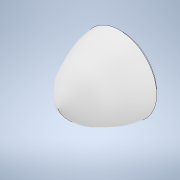
# Autodesk Inventor part: nose
Saved by Autodesk Inventor 2020 (Build 240168000, 168)
## iProperties
Created: 2021-01-23
Part Number: nose
Material: ABS Plastic
Document SubType Name: Modeling
Designer: 0x6f736f646f
Density: 1.06 g/cm^3
Appearance: Smooth - White
Author: 0x6f736f646f
Autodesk Inventor part; units mm, degrees
ref_plane "YZ Plane" through (0, 0, 0) normal (1, 0, 0) x (0, 1, 0)
ref_plane "XZ Plane" through (0, 0, 0) normal (0, 1, 0) x (-1, 0, 0)
ref_plane "XY Plane" through (0, 0, 0) normal (0, 0, 1) x (1, 0, 0)
sketch "Sketch1" plane through (0, 0, 0) normal (1, 0, 0) x (0, 1, 0)
  line L0 (-29, -5) -> (-29.0578, -5)
  line L1 (0, 0) -> (-29, 0)
  line L2 (-25, 0) -> (-25, -2)
  line L3 (-25, -2) -> (-27, -2)
  line L4 (-27, -2) -> (-27, 0)
  line L5 (-27, 0) -> (-29, 0)
  line L6 (-25, 0) -> (-25, 10)
  line L7 (0, 37) -> (0, 48)
  line L8 (-29, 0) -> (-28, 12.123) construction
  line L9 (-28, 12.123) -> (-21.8214, 22.5792) construction
  line L10 (-21.8214, 22.5792) -> (-19.8743, 33.396) construction
  line L11 (-19.8743, 33.396) -> (-11.5338, 39.9891) construction
  line L12 (-11.5338, 39.9891) -> (-5.3798, 46.1599) construction
  line L13 (-5.3798, 46.1599) -> (0, 48) construction
  spline S0 degree 4 poles (-29, 0) (-28, 12.123) (-21.8214, 22.5792) (-19.8743, 33.396) (-11.5338, 39.9891) (-5.3798, 46.1599) (0, 48) knots 1 1 1 1 1 2 3 4 4 4 4 4
  line L14 (-25, 10) -> (-10, 10)
  line L15 (-10, 10) -> (-10, 37)
  line L16 (-10, 37) -> (0, 37)
  line L17 (0, -16.4911) -> (0, 63.9467) projected
  dimension "d25" = 2
  dimension "d26" = 2
  dimension "d27" = 2
  dimension "d29" = 10
  dimension "d31" = 29
  dimension "d32" = 48
  dimension "d33" = 25
  dimension "d34" = 15
  dimension "d35" = 27
  constraints: 22 end point, 4 horizontal, 4 perpendicular, 2 point on line, 1 vertical, 3 other
  measures "d25" distance from line of L1.end L4
  measures "d26" distance of L2.end L3.end
  measures "d27" distance of L3.end L4.end
  measures "d29" distance of L2.start L6.end
  measures "d31" distance of L1.end L1.start
  measures "d32" distance of L1.start L7.end
  measures "d33" distance between parallel lines of L6 L7
  measures "d34" distance of L6.end L14.end
  measures "d35" distance of L14.end L15.end
revolve "Revolution1" add sketch "Sketch1" angle 360 about axis through (0, 0, -10) along (0, 0, 1) contours L2 L3 L4 L1 | L1 S0 L7 L16 L15 L14 L6
body "Solid1"
